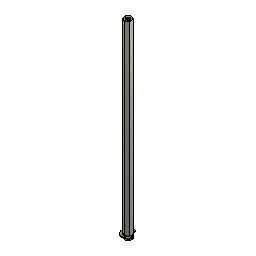
1. Parametric GoBilda REX Shaft (Autodesk Fusion 360 design; units mm, degrees)
Autodesk Fusion 360 part; units mm, degrees
sketch "Sketch1" plane through (0, 0, 0) normal (0, 1, 0) x (1, 0, 0)
  circle A0 centre (0, 0) radius 4
  line L0 (3.5, 2.0207) -> (0, 4.0415)
  line L1 (0, 4.0415) -> (-3.5, 2.0207)
  line L2 (-3.5, 2.0207) -> (-3.5, -2.0207)
  line L3 (-3.5, -2.0207) -> (0, -4.0415)
  line L4 (0, -4.0415) -> (3.5, -2.0207)
  line L5 (3.5, -2.0207) -> (3.5, 2.0207)
  circle A1 centre (0, 0) radius 3
  circle A2 centre (0, 0) radius 2
  dimension "d2" = 8
  dimension "d3" = 3.5
  dimension "d4" = 6
  dimension "d6" = 4
  constraint coincident A0.centre A1.centre
  constraint concentric A1 A2
  measures "d2" diameter of A0
  measures "d3" distance of A0.centre L5
  measures "d4" diameter of A1
  measures "d6" diameter of A2
extrude "Extrude1" add sketch "Sketch1" along normal blind 192 contours A0 L0 L1 L2 L3 L4 L5 | A1 | A2 makes body 1 in component "Shaft"
extrude "Extrude2" cut sketch "Sketch1" along normal blind 10 contours A2 bodies 1 in component "Shaft"
extrude "Extrude3" cut sketch "Sketch1" against normal blind 14 from surface at 192 contours A2 bodies 1 in component "Shaft"
extrude "Extrude4" cut sketch "Sketch1" along normal blind 0.8 from surface at 3.2 contours A0 L0 L1 L2 L3 L4 L5 bodies 1 in component "Shaft"
sketch "Sketch2" plane through (0, 3.2, 0) normal (0, 1, 0) x (-1, 0, 0)
  circle A0 centre (0, 0) radius 3
  arc A1 (-3.4271, 2.0628) -> (-3.5, 1.9365) centre (0, 0) ccw
  line L0 (-3.5, 1.9365) -> (-3.5, -1.9365)
  arc A2 (-3.5, -1.9365) -> (-3.4271, -2.0628) centre (0, 0) ccw
  line L1 (-3.4271, -2.0628) -> (-0.0729, -3.9993)
  arc A3 (-0.0729, -3.9993) -> (0.0729, -3.9993) centre (0, 0) ccw
  line L2 (0.0729, -3.9993) -> (3.4271, -2.0628)
  arc A4 (3.4271, -2.0628) -> (3.5, -1.9365) centre (0, 0) ccw
  line L3 (3.5, -1.9365) -> (3.5, 1.9365)
  arc A5 (3.5, 1.9365) -> (3.4271, 2.0628) centre (0, 0) ccw
  line L4 (3.4271, 2.0628) -> (0.0729, 3.9993)
  arc A6 (0.0729, 3.9993) -> (-0.0729, 3.9993) centre (0, 0) ccw
  line L5 (-0.0729, 3.9993) -> (-3.4271, 2.0628)
  line L6 (-5.3619, 0.9232, 0.8) -> (-2.9326, 0.6323, 0.8)
  arc A7 through (1.8314, 2.3761, 0.8) (2.5532, 1.5751, 0.8) (2.9452, 0.5707, 0.8)
  arc A8 through (-2.9326, 0.6323, 0.8) (-2.45, 1.7313, 0.8) (-1.5751, 2.5532, 0.8)
  line L7 (-1.5751, 2.5532, 0.8) -> (-2.0794, 3.3706, 0.8)
  line L8 (2.4177, 3.1367, 0.8) -> (1.8314, 2.3761, 0.8)
  arc A9 through (4.3864, 0.377, 0.8) (4.0319, -1.7683, 0.8) (2.6938, -3.4823, 0.8)
  arc A10 through (-1.5806, -5.2061, 0.8) (-1.5331, -5.7423, 0.8) (-1.0928, -6.0521, 0.8)
  arc A11 through (2.6938, -3.4823, 0.8) (2.3617, -3.5633, 0.8) (2.0794, -3.3706, 0.8)
  line L9 (2.0794, -3.3706, 0.8) -> (1.5751, -2.5532, 0.8)
  arc A12 through (1.5751, -2.5532, 0.8) (0.4481, -2.9663, 0.8) (-0.7507, -2.9046, 0.8)
  line L10 (2.9452, 0.5707, 0.8) -> (3.8881, 0.7534, 0.8)
  line L11 (-0.7507, -2.9046, 0.8) -> (-1.5806, -5.2061, 0.8)
  arc A13 through (-1.9035, 3.9698, 0.8) (0.2286, 4.3966, 0.8) (2.305, 3.751, 0.8)
  arc A14 through (2.305, 3.751, 0.8) (2.4982, 3.469, 0.8) (2.4177, 3.1367, 0.8)
  arc A15 through (-5.8991, 1.7387, 0.8) (-5.8198, 1.2063, 0.8) (-5.3619, 0.9232, 0.8)
  arc A16 through (-1.0928, -6.0521, 0.8) (5.2341, 3.229, 0.8) (-5.8991, 1.7387, 0.8)
  arc A17 through (-2.0794, 3.3706, 0.8) (-2.1249, 3.7094, 0.8) (-1.9035, 3.9698, 0.8)
  arc A18 through (3.8881, 0.7534, 0.8) (4.2211, 0.6762, 0.8) (4.3864, 0.377, 0.8)
  arc A19 through (2.305, 3.751, 0.8) (2.4982, 3.469, 0.8) (2.4177, 3.1367, 0.8)
  arc A20 through (-1.9035, 3.9698, 0.8) (0.2286, 4.3966, 0.8) (2.305, 3.751, 0.8)
  line L12 (2.4177, 3.1367, 0.8) -> (1.8314, 2.3761, 0.8)
  line L13 (2.0794, -3.3706, 0.8) -> (1.5751, -2.5532, 0.8)
  arc A21 through (3.8881, 0.7534, 0.8) (4.2211, 0.6762, 0.8) (4.3864, 0.377, 0.8)
  arc A22 through (-5.8991, 1.7387, 0.8) (-5.8198, 1.2063, 0.8) (-5.3619, 0.9232, 0.8)
  line L14 (-5.3619, 0.9232, 0.8) -> (-2.9326, 0.6323, 0.8)
  arc A23 through (1.5751, -2.5532, 0.8) (0.4481, -2.9663, 0.8) (-0.7507, -2.9046, 0.8)
  arc A24 through (4.3864, 0.377, 0.8) (4.0319, -1.7683, 0.8) (2.6938, -3.4823, 0.8)
  arc A25 through (-1.0928, -6.0521, 0.8) (5.2341, 3.229, 0.8) (-5.8991, 1.7387, 0.8)
  arc A26 through (-1.5806, -5.2061, 0.8) (-1.5331, -5.7423, 0.8) (-1.0928, -6.0521, 0.8)
  arc A27 through (1.8314, 2.3761, 0.8) (2.5532, 1.5751, 0.8) (2.9452, 0.5707, 0.8)
  line L15 (-1.5751, 2.5532, 0.8) -> (-2.0794, 3.3706, 0.8)
  line L16 (2.9452, 0.5707, 0.8) -> (3.8881, 0.7534, 0.8)
  arc A28 through (-2.0794, 3.3706, 0.8) (-2.1249, 3.7094, 0.8) (-1.9035, 3.9698, 0.8)
  arc A29 through (2.6938, -3.4823, 0.8) (2.3617, -3.5633, 0.8) (2.0794, -3.3706, 0.8)
  arc A30 through (-2.9326, 0.6323, 0.8) (-2.45, 1.7313, 0.8) (-1.5751, 2.5532, 0.8)
  line L17 (-0.7507, -2.9046, 0.8) -> (-1.5806, -5.2061, 0.8)
  line L18 (-1.5806, -5.2061, 0.8) -> (0.3815, 0.2354, 0.8)
  line L19 (-5.3619, 0.9232, 0.8) -> (0.3815, 0.2354, 0.8)
  line L20 (0, 0, 0.8) -> (0.3815, 0.2354, 0.8)
extrude "Extrude1'" add sketch "Sketch2" against normal blind 0.8 separate body contours L6 A7 A8 L7 L8 A9 A10 A11 L9 A12 L10 L11 A13 A14 A15 A16 A17 A18 A19 A20 L12 L13 A21 A22 L14 A23 A24 A25 A26 A27 L15 L16 A28 A29 A30 L17 L18 L19 in plane through (0, 4, 0) normal (0, 1, 0) makes body 2 in component "Clip"
sketch "Sketch1 (2)" plane through (0, 0, 0) normal (0, 0, 1) x (1, 0, 0) in component "Shaft"
  line L0 (-3.4271, 4) -> (-3.5, 4)
  line L1 (-3, 4) -> (-3.4271, 4)
  line L2 (3.4271, 4) -> (3, 4)
  line L3 (3.5, 4) -> (3.4271, 4)
  line L4 (3.4271, 3.2) -> (3.5, 3.2)
  line L5 (3, 3.2) -> (3.4271, 3.2)
  line L6 (-3.4271, 3.2) -> (-3, 3.2)
  line L7 (-3.5, 3.2) -> (-3.4271, 3.2)
  line L8 (-3.5, 0) -> (-3.5, 3.2)
  line L9 (-3.5, 4) -> (-3.5, 192)
  line L10 (-3.4271, 0) -> (-3.5, 0)
  line L11 (-0.0729, 0) -> (-3.4271, 0)
  line L12 (0.0729, 0) -> (-0.0729, 0)
  line L13 (3.4271, 0) -> (0.0729, 0)
  line L14 (3.5, 0) -> (3.5, 3.2)
  line L15 (3.5, 0) -> (3.4271, 0)
  line L16 (-3.4271, 192) -> (-3.5, 192)
  line L17 (-0.0729, 192) -> (-3.4271, 192)
  line L18 (0.0729, 192) -> (-0.0729, 192)
  line L19 (3.4271, 192) -> (0.0729, 192)
  line L20 (3.5, 192) -> (3.4271, 192)
  line L21 (3.5, 4) -> (3.5, 192)
  line L22 (3, 3.2) -> (3, 4)
  line L23 (-3, 3.2) -> (-3, 4)
  line L24 (0, 0) -> (0, -0.15)
  line L25 (0, 0) -> (3.5, 0)
  line L26 (3.5, 0) -> (4, 0)
  line L27 (4, 0) -> (4, 0.5)
  line L28 (4, 0.5) -> (3.5, 0)
  line L29 (4, 0.5) -> (4, 191.5)
  line L30 (4, 191.5) -> (4, 192)
  line L31 (4, 192) -> (3.5, 192)
  line L32 (4, 191.5) -> (3.5, 192)
  dimension "d25" = 3.5
  dimension "d26" = 0.5
  dimension "d27" = 0.5
  dimension "d29" = 191
  dimension "d30" = 0.5
  dimension "d31" = 0.5
  constraint coincident L24.start L25.start
  constraint perpendicular L12 L24
  constraint perpendicular L24 L25
  constraint perpendicular L14 L26
  constraint perpendicular L26 L27
  constraint parallel L27 L29
  constraint parallel L29 L30
  constraint perpendicular L30 L31
  measures "d25" distance of L24.start L14.start
  measures "d26" distance of L14.start L26.end
  measures "d27" distance of L26.end L27.end
  measures "d29" distance of L27.end L29.end
  measures "d30" distance of L29.end L30.end
  measures "d31" distance of L30.end L20.start
revolve "Revolve1" cut sketch "Sketch1 (2)" angle 360 about axis through (0, 0, 0) along (0, -1, 0) contours L30 L31 L32 | L26 L27 L28 bodies 1 in component "Shaft"
thread "Thread3" "ISO Metric profile 4.0 M4x0.7 6H" major diameter 4.1095 minor diameter 3.332 pitch 0.7 angle 60 modelled right hand crest width 0.193 on face at (1.9901, 182.6667, 0.1991) from (0, 192, 0) to (0, 182, 0) crest through (1.666, 191.825, 0) on bodies 1 in component "Shaft"
thread "Thread4" "ISO Metric profile 4.0 M4x0.7 6H" major diameter 4.1095 minor diameter 3.332 pitch 0.7 angle 60 modelled right hand crest width 0.193 on face at (1.9975, 6.6667, 0.0997) from (0, 0, 0) to (0, 10, 0) crest through (1.666, 0.175, 0) on bodies 1 in component "Shaft"
component "Shaft" placed x (1, 0, 0) y (0, 1, 0) z (0, 0, 1) at (0, 0, 0)
component "Clip" placed x (1, 0, 0) y (0, 1, 0) z (0, 0, 1) at (0, 0, 0)
equation "lengthREXShaft = 192 mm"
equation "d3 = ( 7 / 2 ) * 1 mm"
equation "d7 = lengthREXShaft"
equation "d29 = lengthREXShaft - 1 mm"
